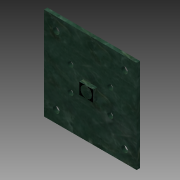
# Autodesk Inventor part: Board
Saved by Autodesk Inventor 2014 (Build 180170000, 170)
## iProperties
Created: 2014-02-09
Part Number: Board
Material: Generic
Document SubType Name: Modeling
Designer: Spooner
Density: 1 g/cm^3
Appearance: Green Polished
Author: Spooner
Autodesk Inventor part; units mm, degrees
ref_plane "YZ Plane" through (0, 0, 0) normal (1, 0, 0) x (0, 1, 0)
ref_plane "XZ Plane" through (0, 0, 0) normal (0, 1, 0) x (-1, 0, 0)
ref_plane "XY Plane" through (0, 0, 0) normal (0, 0, 1) x (1, 0, 0)
sketch "Sketch1" plane through (0, 0, 0) normal (0, 0, 1) x (1, 0, 0)
  line L0 (0, 0) -> (42.0878, 0)
  line L1 (42.0878, 0) -> (42.0878, 42.0878)
  line L2 (42.0878, 42.0878) -> (0, 42.0878)
  line L3 (0, 42.0878) -> (0, 0)
  dimension "d0" = 42.0878
  dimension "d1" = 42.0878
  constraints: 8 end point, 2 parallel, 1 horizontal, 1 perpendicular
  measures "d0" distance of L0.start L0.end
  measures "d1" distance of L2.end L0.start
extrude "Extrusion1" add sketch "Sketch1" along normal blind 1.5748
sketch "Sketch2" plane through (0, 0, 1.5748) normal (0, 0, 1) x (1, 0, 0)
  line L0 (0, 0) -> (42.0878, 0) projected
  line L1 (42.0878, 0) -> (42.0878, 42.0878) projected
  line L2 (42.0878, 42.0878) -> (0, 42.0878) projected
  line L3 (0, 42.0878) -> (0, 0) projected
  circle A0 centre (5.5104, 36.5774) radius 1.5
  circle A1 centre (36.5774, 36.5774) radius 1.5
  circle A2 centre (36.5774, 5.5104) radius 1.5
  circle A3 centre (5.5104, 5.5104) radius 1.5
  circle A4 centre (12.0142, 26.5938) radius 1.2954
  circle A5 centre (30.0736, 26.5938) radius 1.2954
  circle A6 centre (12.0142, 15.494) radius 1.2954
  circle A7 centre (30.0736, 15.494) radius 1.2954
  dimension "d4" = 3
  dimension "d5" = 2.5908
  dimension "d6" = 28.067
  dimension "d7" = 4.0104
  dimension "d8" = 4.0104
  dimension "d9" = 28.067
  dimension "d10" = 4.0104
  dimension "d11" = 15.4686
  dimension "d12" = 8.509
  dimension "d13" = 10.7188
  dimension "d14" = 10.7188
  dimension "d15" = 14.1986
  dimension "d16" = 14.1986
  constraints: 8 centre point, 6 equal radius, 4 horizontal alignment, 4 vertical alignment
  measures "d4" diameter of A0
  measures "d5" diameter of A4
  measures "d7" distance edge to line of A0 L3
  measures "d8" distance edge to line of A1 L1
  measures "d10" distance edge to line of A0 L2
  measures "d13" distance edge to line of A4 L3
  measures "d14" distance edge to line of A5 L1
  measures "d15" distance edge to line of A6 L0
  measures "d16" distance edge to line of A4 L2
extrude "Extrusion2" cut sketch "Sketch2" against normal through all contours A0 | A1 | A2 | A3 | A4 | A5 | A6 | A7
sketch "Sketch3" plane through (0, 0, 1.5748) normal (0, 0, 1) x (1, 0, 0)
  line L0 (0, 0) -> (42.0878, 0) projected
  line L1 (42.0878, 0) -> (42.0878, 42.0878) projected
  line L2 (42.0878, 42.0878) -> (0, 42.0878) projected
  line L3 (0, 42.0878) -> (0, 0) projected
  line L4 (17.8943, 23.622) -> (24.1935, 23.622)
  line L5 (24.1935, 23.622) -> (24.1935, 18.4658)
  line L6 (24.1935, 18.4658) -> (17.8943, 18.4658)
  line L7 (17.8943, 18.4658) -> (17.8943, 23.622)
  dimension "d19" = 6.2992
  dimension "d20" = 5.1562
  dimension "d21" = 18.4658
  dimension "d22" = 18.4658
  dimension "d23" = 17.8943
  dimension "d24" = 17.8943
  constraints: 8 end point, 2 parallel, 1 horizontal, 1 perpendicular
  measures "d19" distance of L5.end L6.end
  measures "d20" distance of L6.end L4.start
  measures "d21" distance between parallel lines of L2 L4
  measures "d22" distance between parallel lines of L0 L6
  measures "d23" distance between parallel lines of L1 L5
  measures "d24" distance between parallel lines of L3 L7
extrude "Extrusion3" add sketch "Sketch3" along normal blind 1.8796 contours L4 L5 L6 L7
sketch "Sketch4" plane through (0, 0, 3.4544) normal (0, 0, 1) x (1, 0, 0)
  line L0 (24.1935, 23.622) -> (17.8943, 23.622) projected
  line L1 (17.8943, 23.622) -> (17.8943, 18.4658) projected
  line L2 (17.8943, 18.4658) -> (24.1935, 18.4658) projected
  line L3 (24.1935, 18.4658) -> (24.1935, 23.622) projected
  circle A0 centre (21.0439, 21.0439) radius 2.5781
  point P0 (0, 0)
  dimension "d27" = 3.1496
  dimension "d28" = 3.1496
  constraints: 2 tangent, 1 centre point
  measures "d27" distance from line of L1 A0.centre
  measures "d28" distance from line of L3 A0.centre
extrude "Extrusion4" add sketch "Sketch4" along normal blind 0.0254 contours A0
equation "\"d1\" = d0"
equation "\"d7\" = d8"
equation "\"d9\" = d6"
equation "\"d10\" = d8"
equation "\"d13\" = d14"
equation "\"d15\" = d16"
equation "\"d21\" = d22"
equation "\"d23\" = d24"
equation "\"d27\" = d28"
body "Solid1"
